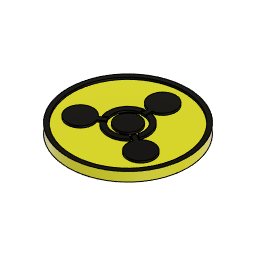
ChemicalCAM (Autodesk Fusion 360 design; units mm, degrees)
Autodesk Fusion 360 part; units mm, degrees
sketch "Sketch1" plane through (0, 0, 0) normal (0, 0, 1) x (1, 0, 0)
  circle A0 centre (0, 0) radius 127
  dimension "d1" = 254
  constraint coincident A0.centre origin
  measures "d1" diameter of A0
extrude "Extrude1" add sketch "Sketch1" along normal blind 15.5
sketch "Sketch3" plane through (0, 0, 15.5) normal (0, 0, 1) x (-1, 0, 0)
  circle A0 centre (0, 0) radius 127
  circle A1 centre (0, 0) radius 25
  circle A2 centre (0, 0) radius 32.5
  circle A3 centre (0, 0) radius 42.5
  line L0 (4.375, -42.2742) -> (-4.375, -42.2742) construction
  line L1 (-4.375, -42.2742) -> (-4.375, -47.2742)
  line L2 (4.375, -42.2742) -> (4.375, -47.2742)
  line L3 (-4.375, -47.2742) -> (4.375, -47.2742) construction
  line L4 (0, -47.2742) -> (0, -73.7742) construction
  circle A4 centre (0, -73.7742) radius 27.5
  line L5 (-4.375, -42.2742) -> (-4.375, -32.2042)
  line L6 (4.375, -42.2742) -> (4.375, -32.2042)
  line L7 (-6.875, -41.9402) -> (-6.875, -31.7645)
  line L8 (-6.875, -41.9402) -> (6.875, -41.9402) construction
  line L9 (6.875, -41.9402) -> (6.875, -31.7645)
  line L10 (-34.423, 24.926) -> (-38.798, 17.3482) construction
  line L11 (-36.6105, 21.1371) -> (0, -42.2742) construction
  line L12 (34.423, 24.926) -> (38.798, 17.3482) construction
  line L13 (36.6105, 21.1371) -> (0, -42.2742) construction
  line L14 (-36.6105, 21.1371) -> (36.6105, 21.1371) construction
  line L15 (-38.798, 17.3482) -> (-30.0771, 12.3132)
  line L16 (-34.423, 24.926) -> (-25.7021, 19.891)
  line L17 (-34.423, 24.926) -> (-30.0929, 22.426)
  line L18 (-38.798, 17.3482) -> (-34.4679, 14.8482)
  circle A5 centre (-64.4531, 37.212) radius 27.5
  line L19 (-39.7588, 15.0162) -> (-32.8838, 26.924) construction
  line L20 (-39.7588, 15.0162) -> (-30.9464, 9.9283)
  line L21 (-32.8838, 26.924) -> (-24.0714, 21.8362)
  line L22 (34.423, 24.926) -> (30.0929, 22.426)
  line L23 (38.798, 17.3482) -> (34.4679, 14.8482)
  circle A6 centre (64.4531, 37.212) radius 27.5
  line L24 (34.423, 24.926) -> (25.7021, 19.891)
  line L25 (38.798, 17.3482) -> (30.0771, 12.3132)
  line L26 (32.8838, 26.924) -> (39.7588, 15.0162) construction
  line L27 (32.8838, 26.924) -> (24.0714, 21.8362)
  line L28 (39.7588, 15.0162) -> (30.9464, 9.9283)
  circle A7 centre (0, 0) radius 118.5
  line L29 (-38.798, 17.3482) -> (-43.1282, 19.8482)
  line L30 (-34.423, 24.926) -> (-38.7532, 27.426)
  line L31 (34.423, 24.926) -> (38.7532, 27.426)
  line L32 (38.798, 17.3482) -> (43.1282, 19.8482)
  line L33 (-43.1282, 19.8482) -> (-38.7532, 27.426) construction
  line L34 (38.7532, 27.426) -> (43.1282, 19.8482) construction
  dimension "d19" = 50
  dimension "d20" = 7.5
  dimension "d21" = 17.5
  dimension "d22" = 8.75
  dimension "d23" = 5
  dimension "d24" = 26.5
  dimension "d25" = 55
  dimension "d26" = 13.75
  dimension "d32" = 237
  dimension "d33" = 5
  dimension "d35" = 5
  constraint concentric A0 A1
  constraint coincident A3 L0.start
  constraint coincident A3 L0.end
  constraint horizontal L0
  constraint perpendicular L0 L1
  constraint perpendicular L0 L2
  constraint equal L1 L2
  constraint midpoint L3 L4.start
  constraint perpendicular L3 L4
  constraint coincident L4.end A4.centre
  constraint coincident A2 L5.end
  constraint perpendicular L0 L5
  constraint coincident A2 L6.end
  constraint perpendicular L0 L6
  constraint coincident A3 L7.start
  constraint coincident A2 L7.end
  constraint parallel L6 L7
  constraint coincident A3 L8.end
  constraint perpendicular L6 L8
  constraint coincident A2 L9.end
  constraint perpendicular L8 L9
  constraint coincident A3 L10.start
  constraint coincident A3 L10.end
  constraint midpoint L10 L11.start
  constraint midpoint L0 L11.end
  constraint coincident A3 L12.start
  constraint coincident A3 L12.end
  constraint equal L0 L12
  constraint midpoint L12 L13.start
  constraint equal L11 L13
  constraint equal L13 L14
  constraint coincident A2 L15.end
  constraint perpendicular L10 L15
  constraint coincident A2 L16.end
  constraint perpendicular L10 L16
  constraint perpendicular L10 L17
  constraint perpendicular L10 L18
  constraint equal L1 L18
  constraint equal L17 L18
  constraint equal A4 A5
  constraint equal L0 L10
  constraint coincident A3 L19.start
  constraint coincident A3 L19.end
  constraint perpendicular L17 L19
  constraint equal L8 L19
  constraint coincident A2 L20.end
  constraint perpendicular L19 L20
  constraint coincident A2 L21.end
  constraint perpendicular L19 L21
  constraint perpendicular L12 L22
  constraint perpendicular L12 L23
  constraint equal L22 L23
  constraint equal L2 L23
  constraint equal A4 A6
  constraint coincident A2 L24.end
  constraint perpendicular L12 L24
  constraint coincident A2 L25.end
  constraint perpendicular L12 L25
  constraint coincident A3 L26.start
  constraint coincident A3 L26.end
  constraint coincident A2 L27.end
  constraint perpendicular L26 L27
  constraint coincident A2 L28.end
  constraint perpendicular L26 L28
  constraint equal L8 L26
  constraint perpendicular L25 L26
  constraint concentric A0 A7
  constraint coincident A5 L29.end
  constraint perpendicular L10 L29
  constraint coincident A5 L30.end
  constraint perpendicular L10 L30
  constraint coincident A6 L31.end
  constraint perpendicular L12 L31
  constraint coincident A6 L32.end
  constraint perpendicular L12 L32
  constraint perpendicular L29 L33
  constraint perpendicular L32 L34
  measures "d19" diameter of A1
  measures "d22" distance of L0.start L0.end
  measures "d23" distance of L0.end L1.end
  measures "d24" distance of L4.start L4.end
  measures "d25" diameter of A4
  measures "d26" distance of L7.start L8.end
  measures "d32" diameter of A7
  measures "d33" distance of L10 L33
  measures "d35" distance of L12 L34
extrude "Extrude3" add sketch "Sketch3" along normal blind 4 contours A0 | A1 | A2 A3 L9 L28 | A2 A3 L22 L23 L24 L25 | A2 A3 L5 L6 | A3 A6 L31 L32 | A3 L1 L2 A4 | A2 A3 L21 L27 | A6 | A2 A3 L7 L20 | A4 | A2 A3 L15 L16 L17 L18 | A3 A5 L29 L30 | A5
